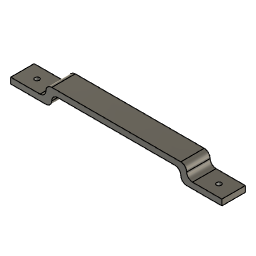
bin handle v1 (Autodesk Fusion 360 design; units mm, degrees)
Autodesk Fusion 360 part; units mm, degrees
note: some values were not read from the file. Set by a fixed rule: which sketch regions a step uses.
sketch "Sketch5" plane through (0, 0, 0) normal (0, 1, 0) x (1, 0, 0) in component "bin handle"
  line L0 (0, 0) -> (30, 0)
  line L1 (25, -5) -> (0, -5)
  line L2 (0, -5) -> (0, 0)
  arc A0 (30, -10) -> (25, -5) centre (25, -10) ccw
  arc A1 (35, -5) -> (29.9988, 0) centre (30, -5) ccw
  arc A2 (29.9997, -9.9447) -> (35.0276, -15.0005) centre (35, -10) ccw
  arc A3 (35, -5) -> (40.0006, -10) centre (40, -5) ccw
  line L3 (40.0006, -15.0005) -> (35, -15.0005)
  line L4 (40.0006, -10) -> (40.0006, -10.0005)
  arc A4 (145, -5) -> (150.0012, 0) centre (150, -5) cw
  arc A5 (145, -5) -> (139.9994, -10) centre (140, -5) cw
  line L5 (139.9994, -10) -> (139.9994, -10.0005)
  line L6 (180, -5) -> (180, 0)
  line L7 (180, 0) -> (150, 0)
  arc A6 (150.0003, -9.9447) -> (144.9724, -15.0005) centre (145, -10) cw
  arc A7 (150, -10) -> (155, -5) centre (155, -10) cw
  line L8 (139.9994, -15.0005) -> (145, -15.0005)
  line L9 (155, -5) -> (180, -5)
  line L10 (139.9994, -10.0005) -> (139.9994, -10)
  line L11 (40.0006, -10) -> (40.0006, -10.0005)
  line L12 (40.0006, -15.0005) -> (140.0006, -15.0005)
  line L13 (140.0006, -10.0005) -> (40.0006, -10.0005)
  spline S0 degree 5 poles (145, -15.0005) (145.3487, -15.0005) (146.0192, -14.9475) (146.9445, -14.7088) (148.0257, -14.1119) (149.1116, -13.0258) (149.7083, -11.9445) (149.9469, -11.0192) (150, -10.3487) (150, -10) knots 0 0 0 0 0 0 0.2 0.4 0.6 0.8 1 1 1 1 1 1
  point P0 (180, 0)
  dimension "d22" = 35
  dimension "d23" = 35
  dimension "d25" = 100
  constraint horizontal L0
  constraint horizontal L1
  constraint vertical L2
  constraint coincident L0.start L2.end
  constraint coincident L0 A1.end
  constraint coincident A0 A2.start
  constraint horizontal L3
  constraint coincident L3 A2.end
  constraint perpendicular L3 L4
  constraint coincident P0 L6.end
  constraint coincident A4.end L7
  constraint coincident A6.start A7
  constraint coincident A6.end L8
  constraint perpendicular L5 L8
  constraint vertical L10
  constraint vertical L11
  constraint horizontal L12
  constraint horizontal L13
  constraint coincident L13 L5.end
  constraint tangent A7 S0
  measures "d22" horizontal distance of L0.start A1.start
  measures "d23" horizontal distance of P0 A4.start
  measures "d25" distance of L3.start L12.end
extrude "Extrude2" add sketch "Sketch5" along normal blind 20 in component "bin handle"
sketch "Sketch6" plane through (0, 0, 5) normal (0, 0, 1) x (-1, 0, 0) in component "bin handle"
  line L0 (0, 0) -> (-25, 0)
  line L1 (-25, 0) -> (-25, -20)
  line L2 (-25, -20) -> (0, -20)
  line L3 (0, -20) -> (0, 0)
  circle A0 centre (-12.5, -10) radius 2
  dimension "d29" = 4
  measures "d29" diameter of A0
sketch "Sketch7" plane through (0, 0, 5) normal (0, 0, 1) x (-1, 0, 0) in component "bin handle"
  line L0 (-155, 0) -> (-180, 0)
  line L1 (-180, 0) -> (-180, -20)
  line L2 (-180, -20) -> (-155, -20)
  line L3 (-155, -20) -> (-155, 0)
  circle A0 centre (-167.5, -10) radius 2
  dimension "d30" = 4
  measures "d30" diameter of A0
hole "Hole1" at (167.5, 10, 5) direction (0, 0, -1) diameter 4 depth 5 tip angle 118 in component "bin handle"
hole "Hole2" at (12.5, 10, 5) direction (0, 0, -1) diameter 4 depth 5 tip angle 118 in component "bin handle"
component "bin handle" placed x (1, 0, 0) y (0, 1, 0) z (0, 0, 1) at (0, 0, 0)
